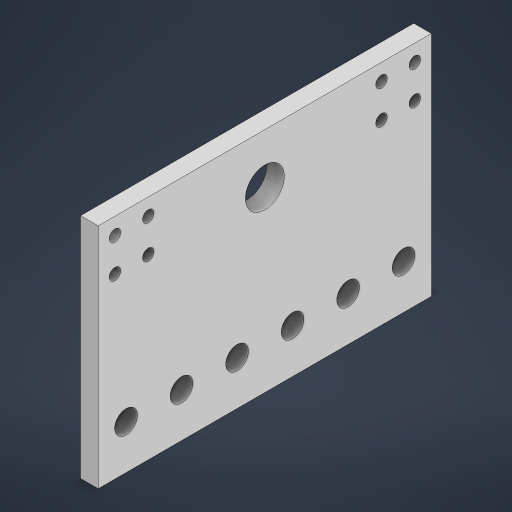
# Autodesk Inventor part: ArmSupportPlate
Saved by Autodesk Inventor 2024 (Build 280153000, 153)
## iProperties
Created: 2024-01-05
Part Number: ArmSupportPlate
Material: Generic
Document SubType Name: Modeling
Designer: avsar
Density: 1 g/cm^3
Appearance: Default
Author: avsar
Autodesk Inventor part; units mm, degrees
ref_plane "YZ Plane" through (0, 0, 0) normal (1, 0, 0) x (0, 1, 0)
ref_plane "XZ Plane" through (0, 0, 0) normal (0, 1, 0) x (-1, 0, 0)
ref_plane "XY Plane" through (0, 0, 0) normal (0, 0, 1) x (1, 0, 0)
sketch "Sketch1" plane through (0, 0, 0) normal (1, 0, 0) x (0, 1, 0)
  line L0 (-41, 60) -> (41, 60)
  line L1 (41, 60) -> (41, -60)
  line L2 (41, -60) -> (-41, -60)
  line L3 (-41, -60) -> (-41, 60)
  line L4 (-41, 60) -> (41, -60) construction
  line L5 (41, 60) -> (-41, -60) construction
  point P0 (0, 0)
  dimension "d0" = 82
  dimension "d1" = 120
  constraints: 12 end point, 2 midpoint, 2 parallel, 1 horizontal, 1 perpendicular
  measures "d0" distance of L1.end L2.end
  measures "d1" distance of L0.end L1.end
extrude "Extrusion1" add sketch "Sketch1" along normal blind 6.35
sketch "Sketch2" plane through (6.35, 0, 0) normal (1, 0, 0) x (0, 0, -1)
  circle A0 centre (-50, -25.125) radius 4.1
  line L0 (-60, -41) -> (60, -41) construction
  circle A1 centre (-30, -25.125) radius 4.1
  circle A2 centre (-10, -25.125) radius 4.1
  circle A3 centre (10, -25.125) radius 4.1
  circle A4 centre (30, -25.125) radius 4.1
  circle A5 centre (50, -25.125) radius 4.1
  point P0 (0, 0)
  dimension "d4" = 8.2
  dimension "d5" = 15.875
  dimension "d6" = 50
  dimension "d9" = 20
  constraints: 6 centre point, 1 horizontal, 10 other
  measures "d4" diameter of A0
  measures "d5" distance from line of L0 A0.centre
  measures "d6" horizontal distance of point (0, 0) A0.centre
  measures "d9" distance of A0.centre A1.centre
extrude "Extrusion2" cut sketch "Sketch2" against normal through all
sketch "Sketch3" plane through (6.35, 0, 0) normal (1, 0, 0) x (0, 0, -1)
  circle A0 centre (0, 23) radius 7
  line L0 (-60, -41) -> (60, -41) projected
  point P0 (0, 0)
  point P1 (0, -41)
  dimension "d16" = 14
  dimension "d17" = 64
  constraints: 1 centre point, 1 midpoint, 1 vertical alignment
  measures "d16" diameter of A0
  measures "d17" distance of point (0, -41) A0.centre
extrude "Extrusion3" cut sketch "Sketch3" against normal through all
sketch "Sketch4" plane through (6.35, 0, 0) normal (1, 0, 0) x (0, 0, -1)
  circle A0 centre (-48, 29) radius 2.5 construction
  circle A1 centre (-54, 35) radius 2.05
  circle A2 centre (-54, 23) radius 2.05
  circle A3 centre (-42, 23) radius 2.05
  circle A4 centre (-42, 35) radius 2.05
  line L0 (-60, 41) -> (-60, -41) projected
  line L1 (60, 41) -> (-60, 41) projected
  circle A5 centre (0, 23) radius 7 projected
  line L2 (0, 30) -> (0, 15.8616) construction
  circle A6 centre (48, 29) radius 2.5 construction
  circle A7 centre (54, 35) radius 2.05
  circle A8 centre (54, 23) radius 2.05
  circle A9 centre (42, 23) radius 2.05
  circle A10 centre (42, 35) radius 2.05
  line L3 (60, 41) -> (60, -41)
  line L4 (-60, 41) -> (60, 41)
  point P0 (0, 0)
  dimension "d20" = 5
  dimension "d21" = 4.1
  dimension "d22" = 6
  dimension "d23" = 6
  dimension "d26" = 360
  dimension "d28" = 12
  dimension "d29" = 12
  constraints: 10 centre point, 8 symmetric about line, 6 end point, 1 point on line, 1 vertical, 1 vertical alignment, 15 other
  measures "d20" diameter of A0
  measures "d21" diameter of A1
  measures "d22" horizontal distance of A0.centre A1.centre
  measures "d23" horizontal distance of A0.centre A1.centre
  measures "d28" distance from line of L0 A0.centre
  measures "d29" distance from line of L1 A0.centre
extrude "Extrusion4" cut sketch "Sketch4" against normal through all contours A1 | A2 | A3 | A4 | A7 | A8 | A9 | A10
body "Solid1"
